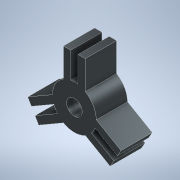
# Autodesk Inventor part: Rotor
Saved by Autodesk Inventor 2022.1 (Build 261234020, 234B)
## iProperties
Created: 2023-07-21
Part Number: Rotor
Material: Iron, Gray
Document SubType Name: Modeling
Designer: SENAI
Mass: 493.198 g
Surface Area: 193.17 cm^2
Volume: 68.9787 cm^3
Density: 7.15 g/cm^3
Appearance: Iron Gray
Author: SENAI
Autodesk Inventor part; units mm, degrees
ref_plane "YZ Plane" through (0, 0, 0) normal (1, 0, 0) x (0, 1, 0)
ref_plane "XZ Plane" through (0, 0, 0) normal (0, 1, 0) x (-1, 0, 0)
ref_plane "XY Plane" through (0, 0, 0) normal (0, 0, 1) x (1, 0, 0)
sketch "Sketch1" plane through (0, 0, 0) normal (0, 0, 1) x (1, 0, 0)
  circle A0 centre (21.3984, 18.434) radius 21
  circle A1 centre (21.3984, 18.434) radius 7.5
  point P0 (0, 0)
  dimension "d0" = 42
  dimension "d1" = 15
  constraints: 2 centre point, 1 coincident
  measures "d0" diameter of A0
  measures "d1" diameter of A1
extrude "Extrusion1" add sketch "Sketch1" along normal blind 30
sketch "Sketch2" plane through (21.3984, 18.434, 30) normal (0, 0, 1) x (1, 0, 0)
  circle A0 centre (0, 0) radius 21 projected
  line L0 (-10.5244, 16.6581) -> (-10.5244, 45.6581)
  line L1 (-10.5244, 45.6581) -> (-3.5244, 45.6581)
  line L2 (-3.5244, 45.6581) -> (-3.5244, 16.6581)
  line L3 (-3.5244, 16.6581) -> (3.4756, 16.6581)
  line L4 (3.4756, 16.6581) -> (3.4756, 45.6581)
  line L5 (3.4756, 45.6581) -> (10.4756, 45.6581)
  line L6 (10.4756, 45.6581) -> (10.4756, 16.6581)
  line L7 (10.4756, 16.6581) -> (-10.5244, 16.6581)
  line L8 (-9.1375, -17.4281) -> (-34.2309, -31.9649)
  line L9 (-34.2309, -31.9649) -> (-37.7398, -25.9078)
  line L10 (-37.7398, -25.9078) -> (-12.6464, -11.371)
  line L11 (-12.6464, -11.371) -> (-16.1552, -5.314)
  line L12 (-16.1552, -5.314) -> (-41.2487, -19.8508)
  line L13 (-41.2487, -19.8508) -> (-44.7576, -13.7938)
  line L14 (-44.7576, -13.7938) -> (-19.6641, 0.7431)
  line L15 (-19.6641, 0.7431) -> (-9.1375, -17.4281)
  line L16 (19.6619, 0.8008) -> (44.7979, -13.6624)
  line L17 (44.7979, -13.6624) -> (41.3067, -19.7297)
  line L18 (41.3067, -19.7297) -> (16.1708, -5.2666)
  line L19 (16.1708, -5.2666) -> (12.6797, -11.3339)
  line L20 (12.6797, -11.3339) -> (37.8156, -25.797)
  line L21 (37.8156, -25.797) -> (34.3245, -31.8643)
  line L22 (34.3245, -31.8643) -> (9.1886, -17.4012)
  line L23 (9.1886, -17.4012) -> (19.6619, 0.8008)
  point P0 (-21.3984, -18.434)
  point P1 (14.4252, -8.3002)
  point P2 (16.1708, -5.2666)
  point P3 (12.6797, -11.3339)
  point P4 (-16.1552, -5.314)
  point P5 (-3.5244, 16.6581)
  point P6 (3.4756, 16.6581)
  dimension "d6" = 29
  dimension "d7" = 7
  dimension "d8" = 29
  dimension "d9" = 7
  dimension "d10" = 29
  dimension "d11" = 7
  dimension "d12" = 29
  dimension "d13" = 45.6581
  dimension "d14" = 3.5244
  dimension "d15" = 29
  dimension "d16" = 7
  dimension "d17" = 29
  dimension "d18" = 7
  dimension "d19" = 29
  dimension "d20" = 7
  dimension "d21" = 29
  dimension "d26" = 29
  dimension "d27" = 7
  dimension "d28" = 29
  dimension "d29" = 7
  dimension "d30" = 29
  dimension "d31" = 7
  dimension "d32" = 29
  dimension "d33" = 29.916
  dimension "d34" = 30.084
  dimension "d35" = 34.3223
  dimension "d36" = 59.3205
  dimension "d37" = 44.8708
  dimension "d38" = 30.163
  constraints: 48 end point, 12 perpendicular, 9 point on line, 1 midpoint, 1 vertical
  measures "d6" distance of L0.start L0.end
  measures "d7" distance of L0.end L1.end
  measures "d8" distance of L1.end L2.end
  measures "d9" distance of L2.end L3.end
  measures "d10" distance of L3.end L4.end
  measures "d11" distance of L4.end L5.end
  measures "d12" distance of L5.end L6.end
  measures "d13" distance from line of A0.centre L1
  measures "d14" distance from line of A0.centre L2
  measures "d15" distance of L8.start L8.end
  measures "d16" distance of L8.end L9.end
  measures "d17" distance of L9.end L10.end
  measures "d18" distance of L10.end L11.end
  measures "d19" distance of L11.end L12.end
  measures "d20" distance of L12.end L13.end
  measures "d21" distance of L13.end L14.end
  measures "d26" distance of L16.start L16.end
  measures "d27" distance of L16.end L17.end
  measures "d28" distance of L17.end L18.end
  measures "d29" distance of L18.end L19.end
  measures "d30" distance of L19.end L20.end
  measures "d31" distance of L20.end L22.start
  measures "d32" distance of L22.start L23.start
  measures "d33" angle of L21 L6
  measures "d34" angle of L6 L15
  measures "d35" distance from line of L16.end L6
  measures "d36" distance from line of L16.end L5
  measures "d37" distance from line of L8.start L17
  measures "d38" distance from line of L8.start L16
extrude "Extrusion2" add sketch "Sketch2" against normal blind 30 contours A0 L18 L23 L16 | A0 L16 L17 L18 | L6 L7 L4 A0 | A0 L4 L5 L6 | L20 L21 L22 A0 | A0 L22 L23 L20 | L2 L7 L0 A0 | A0 L0 L1 L2 | L8 L9 L10 A0 | A0 L10 L15 L8 | L14 L15 L12 A0 | A0 L12 L13 L14
body "Solid1"
